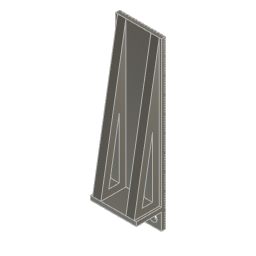
Fixture (Autodesk Fusion 360 design; units mm, degrees)
Autodesk Fusion 360 part; units mm, degrees
(part 1 of 2)
sketch "Sketch1" plane through (0, 0, 0) normal (0, 1, 0) x (1, 0, 0)
  line L0 (0, 0) -> (69.85, 0)
  line L1 (69.85, 0) -> (69.85, -25.4)
  line L2 (69.85, -25.4) -> (0, -25.4)
  line L3 (0, -25.4) -> (0, 0)
  line L4 (4.7498, -25.4) -> (5.5372, -25.4)
  line L5 (5.5372, 0) -> (4.7498, 0)
  line L6 (69.85, -22.225) -> (69.85, -21.4376)
  line L7 (0, -21.4376) -> (0, -22.225)
  line L8 (0, -22.225) -> (4.7498, -22.225)
  line L9 (4.7498, -21.4376) -> (0, -21.4376)
  line L10 (0, -19.05) -> (4.7498, -19.05)
  line L11 (4.7498, -18.2626) -> (0, -18.2626)
  line L12 (0, -15.875) -> (4.7498, -15.875)
  line L13 (4.7498, -15.0876) -> (0, -15.0876)
  line L14 (4.7498, -11.9126) -> (0, -11.9126)
  line L15 (0, -12.7) -> (4.7498, -12.7)
  line L16 (0, -9.525) -> (4.7498, -9.525)
  line L17 (4.7498, -8.7376) -> (0, -8.7376)
  line L18 (0, -6.35) -> (4.7498, -6.35)
  line L19 (4.7498, -5.5626) -> (0, -5.5626)
  line L20 (0, -3.175) -> (4.7498, -3.175)
  line L21 (4.7498, -2.3876) -> (0, -2.3876)
  line L22 (9.4996, -2.3876) -> (5.5372, -2.3876)
  line L23 (5.5372, -3.175) -> (9.4996, -3.175)
  line L24 (9.4996, -5.5626) -> (5.5372, -5.5626)
  line L25 (5.5372, -6.35) -> (9.4996, -6.35)
  line L26 (9.4996, -8.7376) -> (5.5372, -8.7376)
  line L27 (5.5372, -9.525) -> (9.4996, -9.525)
  line L28 (9.4996, -11.9126) -> (5.5372, -11.9126)
  line L29 (5.5372, -12.7) -> (9.4996, -12.7)
  line L30 (9.4996, -15.0876) -> (5.5372, -15.0876)
  line L31 (5.5372, -15.875) -> (9.4996, -15.875)
  line L32 (9.4996, -18.2626) -> (5.5372, -18.2626)
  line L33 (5.5372, -19.05) -> (9.4996, -19.05)
  line L34 (9.4996, -21.4376) -> (5.5372, -21.4376)
  line L35 (5.5372, -22.225) -> (9.4996, -22.225)
  line L36 (10.287, -22.225) -> (14.2494, -22.225)
  line L37 (14.2494, -21.4376) -> (10.287, -21.4376)
  line L38 (10.287, -19.05) -> (14.2494, -19.05)
  line L39 (14.2494, -18.2626) -> (10.287, -18.2626)
  line L40 (10.287, -15.875) -> (14.2494, -15.875)
  line L41 (14.2494, -15.0876) -> (10.287, -15.0876)
  line L42 (10.287, -12.7) -> (14.2494, -12.7)
  line L43 (14.2494, -11.9126) -> (10.287, -11.9126)
  line L44 (10.287, -9.525) -> (14.2494, -9.525)
  line L45 (14.2494, -8.7376) -> (10.287, -8.7376)
  line L46 (10.287, -6.35) -> (14.2494, -6.35)
  line L47 (14.2494, -5.5626) -> (10.287, -5.5626)
  line L48 (10.287, -3.175) -> (14.2494, -3.175)
  line L49 (14.2494, -2.3876) -> (10.287, -2.3876)
  line L50 (18.9992, -2.3876) -> (15.0368, -2.3876)
  line L51 (15.0368, -3.175) -> (18.9992, -3.175)
  line L52 (18.9992, -5.5626) -> (15.0368, -5.5626)
  line L53 (15.0368, -6.35) -> (18.9992, -6.35)
  line L54 (18.9992, -8.7376) -> (15.0368, -8.7376)
  line L55 (15.0368, -9.525) -> (18.9992, -9.525)
  line L56 (18.9992, -11.9126) -> (15.0368, -11.9126)
  line L57 (15.0368, -12.7) -> (18.9992, -12.7)
  line L58 (15.0368, -15.875) -> (18.9992, -15.875)
  line L59 (18.9992, -15.0876) -> (15.0368, -15.0876)
  line L60 (18.9992, -18.2626) -> (15.0368, -18.2626)
  line L61 (15.0368, -19.05) -> (18.9992, -19.05)
  line L62 (18.9992, -21.4376) -> (15.0368, -21.4376)
  line L63 (15.0368, -22.225) -> (18.9992, -22.225)
  line L64 (19.7866, -22.225) -> (23.749, -22.225)
  line L65 (23.749, -21.4376) -> (19.7866, -21.4376)
  line L66 (19.7866, -19.05) -> (23.749, -19.05)
  line L67 (23.749, -18.2626) -> (19.7866, -18.2626)
  line L68 (19.7866, -15.875) -> (23.749, -15.875)
  line L69 (23.749, -15.0876) -> (19.7866, -15.0876)
  line L70 (19.7866, -12.7) -> (23.749, -12.7)
  line L71 (23.749, -11.9126) -> (19.7866, -11.9126)
  line L72 (19.7866, -9.525) -> (23.749, -9.525)
  line L73 (23.749, -8.7376) -> (19.7866, -8.7376)
  line L74 (19.7866, -6.35) -> (23.749, -6.35)
  line L75 (23.749, -5.5626) -> (19.7866, -5.5626)
  line L76 (19.7866, -3.175) -> (23.749, -3.175)
  line L77 (23.749, -2.3876) -> (19.7866, -2.3876)
  line L78 (28.4988, -2.3876) -> (24.5364, -2.3876)
  line L79 (24.5364, -3.175) -> (28.4988, -3.175)
  line L80 (28.4988, -5.5626) -> (24.5364, -5.5626)
  line L81 (24.5364, -6.35) -> (28.4988, -6.35)
  line L82 (28.4988, -8.7376) -> (24.5364, -8.7376)
  line L83 (24.5364, -9.525) -> (28.4988, -9.525)
  line L84 (28.4988, -11.9126) -> (24.5364, -11.9126)
  line L85 (24.5364, -12.7) -> (28.4988, -12.7)
  line L86 (28.4988, -15.0876) -> (24.5364, -15.0876)
  line L87 (24.5364, -15.875) -> (28.4988, -15.875)
  line L88 (28.4988, -18.2626) -> (24.5364, -18.2626)
  line L89 (24.5364, -19.05) -> (28.4988, -19.05)
  line L90 (28.4988, -21.4376) -> (24.5364, -21.4376)
  line L91 (24.5364, -22.225) -> (28.4988, -22.225)
  line L92 (29.2862, -22.225) -> (33.2486, -22.225)
  line L93 (33.2486, -21.4376) -> (29.2862, -21.4376)
  line L94 (29.2862, -19.05) -> (33.2486, -19.05)
  line L95 (33.2486, -18.2626) -> (29.2862, -18.2626)
  line L96 (29.2862, -15.875) -> (33.2486, -15.875)
  line L97 (33.2486, -15.0876) -> (29.2862, -15.0876)
  line L98 (29.2862, -12.7) -> (33.2486, -12.7)
  line L99 (33.2486, -11.9126) -> (29.2862, -11.9126)
  line L100 (29.2862, -9.525) -> (33.2486, -9.525)
  line L101 (33.2486, -8.7376) -> (29.2862, -8.7376)
  line L102 (29.2862, -6.35) -> (33.2486, -6.35)
  line L103 (33.2486, -5.5626) -> (29.2862, -5.5626)
  line L104 (29.2862, -3.175) -> (33.2486, -3.175)
  line L105 (33.2486, -2.3876) -> (29.2862, -2.3876)
  line L106 (37.9984, -2.3876) -> (34.036, -2.3876)
  line L107 (34.036, -3.175) -> (37.9984, -3.175)
  line L108 (37.9984, -5.5626) -> (34.036, -5.5626)
  line L109 (34.036, -6.35) -> (37.9984, -6.35)
  line L110 (37.9984, -8.7376) -> (34.036, -8.7376)
  line L111 (34.036, -9.525) -> (37.9984, -9.525)
  line L112 (37.9984, -11.9126) -> (34.036, -11.9126)
  line L113 (34.036, -12.7) -> (37.9984, -12.7)
  line L114 (37.9984, -15.0876) -> (34.036, -15.0876)
  line L115 (34.036, -15.875) -> (37.9984, -15.875)
  line L116 (37.9984, -18.2626) -> (34.036, -18.2626)
  line L117 (34.036, -19.05) -> (37.9984, -19.05)
  line L118 (37.9984, -21.4376) -> (34.036, -21.4376)
  line L119 (34.036, -22.225) -> (37.9984, -22.225)
  line L120 (38.7858, -22.225) -> (42.7482, -22.225)
  line L121 (42.7482, -21.4376) -> (38.7858, -21.4376)
  line L122 (38.7858, -19.05) -> (42.7482, -19.05)
  line L123 (42.7482, -18.2626) -> (38.7858, -18.2626)
  line L124 (38.7858, -15.875) -> (42.7482, -15.875)
  line L125 (42.7482, -15.0876) -> (38.7858, -15.0876)
  line L126 (38.7858, -12.7) -> (42.7482, -12.7)
  line L127 (42.7482, -11.9126) -> (38.7858, -11.9126)
  line L128 (38.7858, -9.525) -> (42.7482, -9.525)
  line L129 (42.7482, -8.7376) -> (38.7858, -8.7376)
  line L130 (38.7858, -3.175) -> (42.7482, -3.175)
  line L131 (42.7482, -2.3876) -> (38.7858, -2.3876)
  line L132 (42.7482, -5.5626) -> (38.7858, -5.5626)
  line L133 (38.7858, -6.35) -> (42.7482, -6.35)
  line L134 (43.5356, -22.225) -> (47.498, -22.225)
  line L135 (47.498, -21.4376) -> (43.5356, -21.4376)
  line L136 (43.5356, -19.05) -> (47.498, -19.05)
  line L137 (47.498, -18.2626) -> (43.5356, -18.2626)
  line L138 (43.5356, -15.875) -> (47.498, -15.875)
  line L139 (47.498, -15.0876) -> (43.5356, -15.0876)
  line L140 (43.5356, -12.7) -> (47.498, -12.7)
  line L141 (47.498, -11.9126) -> (43.5356, -11.9126)
  line L142 (43.5356, -9.525) -> (47.498, -9.525)
  line L143 (47.498, -8.7376) -> (43.5356, -8.7376)
  line L144 (43.5356, -6.35) -> (47.498, -6.35)
  line L145 (47.498, -5.5626) -> (43.5356, -5.5626)
  line L146 (43.5356, -3.175) -> (47.498, -3.175)
  line L147 (47.498, -2.3876) -> (43.5356, -2.3876)
  line L148 (52.2478, -2.3876) -> (48.2854, -2.3876)
  line L149 (48.2854, -3.175) -> (52.2478, -3.175)
  line L150 (52.2478, -5.5626) -> (48.2854, -5.5626)
  line L151 (48.2854, -6.35) -> (52.2478, -6.35)
  line L152 (52.2478, -8.7376) -> (48.2854, -8.7376)
  line L153 (48.2854, -9.525) -> (52.2478, -9.525)
  line L154 (52.2478, -11.9126) -> (48.2854, -11.9126)
  line L155 (48.2854, -12.7) -> (52.2478, -12.7)
  line L156 (52.2478, -15.0876) -> (48.2854, -15.0876)
  line L157 (48.2854, -15.875) -> (52.2478, -15.875)
  line L158 (52.2478, -18.2626) -> (48.2854, -18.2626)
  line L159 (48.2854, -19.05) -> (52.2478, -19.05)
  line L160 (52.2478, -21.4376) -> (48.2854, -21.4376)
  line L161 (48.2854, -22.225) -> (52.2478, -22.225)
  line L162 (53.0352, -22.225) -> (56.9976, -22.225)
  line L163 (56.9976, -21.4376) -> (53.0352, -21.4376)
  line L164 (53.0352, -19.05) -> (56.9976, -19.05)
  line L165 (56.9976, -18.2626) -> (53.0352, -18.2626)
  line L166 (53.0352, -15.875) -> (56.9976, -15.875)
  line L167 (56.9976, -15.0876) -> (53.0352, -15.0876)
  line L168 (53.0352, -12.7) -> (56.9976, -12.7)
  line L169 (56.9976, -11.9126) -> (53.0352, -11.9126)
  line L170 (53.0352, -9.525) -> (56.9976, -9.525)
  line L171 (56.9976, -9.525) -> (56.9976, -11.9126)
  line L172 (57.785, -11.9126) -> (57.785, -9.525)
  line L173 (56.9976, -8.7376) -> (53.0352, -8.7376)
  line L174 (53.0352, -6.35) -> (56.9976, -6.35)
  line L175 (56.9976, -5.5626) -> (53.0352, -5.5626)
  line L176 (53.0352, -3.175) -> (56.9976, -3.175)
  line L177 (56.9976, -2.3876) -> (53.0352, -2.3876)
  line L178 (61.7474, -2.3876) -> (57.785, -2.3876)
  line L179 (57.785, -3.175) -> (61.7474, -3.175)
  line L180 (61.7474, -5.5626) -> (57.785, -5.5626)
  line L181 (57.785, -6.35) -> (61.7474, -6.35)
  line L182 (61.7474, -8.7376) -> (57.785, -8.7376)
  line L183 (57.785, -9.525) -> (61.7474, -9.525)
  line L184 (61.7474, -11.9126) -> (57.785, -11.9126)
  line L185 (57.785, -12.7) -> (61.7474, -12.7)
  line L186 (61.7474, -15.0876) -> (57.785, -15.0876)
  line L187 (57.785, -15.875) -> (61.7474, -15.875)
  line L188 (61.7474, -18.2626) -> (57.785, -18.2626)
  line L189 (57.785, -19.05) -> (61.7474, -19.05)
  line L190 (61.7474, -21.4376) -> (57.785, -21.4376)
  line L191 (57.785, -22.225) -> (61.7474, -22.225)
  line L192 (62.5348, -22.225) -> (66.4972, -22.225)
  line L193 (67.2846, -22.225) -> (69.85, -22.225)
  line L194 (69.85, -21.4376) -> (67.2846, -21.4376)
  line L195 (66.4972, -21.4376) -> (62.5348, -21.4376)
  line L196 (62.5348, -19.05) -> (66.4972, -19.05)
  line L197 (67.2846, -19.05) -> (69.85, -19.05)
  line L198 (69.85, -18.2626) -> (67.2846, -18.2626)
  line L199 (66.4972, -18.2626) -> (62.5348, -18.2626)
  line L200 (62.5348, -15.875) -> (66.4972, -15.875)
  line L201 (67.2846, -15.875) -> (69.85, -15.875)
  line L202 (69.85, -15.0876) -> (67.2846, -15.0876)
  line L203 (66.4972, -15.0876) -> (62.5348, -15.0876)
  line L204 (62.5348, -12.7) -> (66.4972, -12.7)
  line L205 (67.2846, -12.7) -> (69.85, -12.7)
  line L206 (69.85, -11.9126) -> (67.2846, -11.9126)
  line L207 (66.4972, -11.9126) -> (62.5348, -11.9126)
  line L208 (62.5348, -9.525) -> (66.4972, -9.525)
  line L209 (67.2846, -9.525) -> (69.85, -9.525)
  line L210 (69.85, -8.7376) -> (67.2846, -8.7376)
  line L211 (66.4972, -8.7376) -> (62.5348, -8.7376)
  line L212 (62.5348, -6.35) -> (66.4972, -6.35)
  line L213 (67.2846, -6.35) -> (69.85, -6.35)
  line L214 (69.85, -5.5626) -> (67.2846, -5.5626)
  line L215 (66.4972, -5.5626) -> (62.5348, -5.5626)
  line L216 (62.5348, -3.175) -> (66.4972, -3.175)
  line L217 (67.2846, -3.175) -> (69.85, -3.175)
  line L218 (69.85, -2.3876) -> (67.2846, -2.3876)
  line L219 (66.4972, -2.3876) -> (62.5348, -2.3876)
  line L220 (67.2846, -2.3876) -> (67.2846, 0)
  line L221 (66.4972, 0) -> (66.4972, -2.3876)
  line L222 (62.5348, -2.3876) -> (62.5348, 0)
  line L223 (61.7474, 0) -> (61.7474, -2.3876)
  line L224 (57.785, -2.3876) -> (57.785, 0)
  line L225 (56.9976, 0) -> (56.9976, -2.3876)
  line L226 (56.9976, -3.175) -> (56.9976, -8.7376)
  line L227 (53.0352, -2.3876) -> (53.0352, 0)
  line L228 (52.2478, 0) -> (52.2478, -2.3876)
  line L229 (48.2854, -2.3876) -> (48.2854, 0)
  line L230 (47.498, 0) -> (47.498, -2.3876)
  line L231 (43.5356, -2.3876) -> (43.5356, 0)
  line L232 (42.7482, 0) -> (42.7482, -2.3876)
  line L233 (38.7858, -2.3876) -> (38.7858, 0)
  line L234 (37.9984, 0) -> (37.9984, -2.3876)
  line L235 (34.036, -2.3876) -> (34.036, 0)
  line L236 (33.2486, 0) -> (33.2486, -2.3876)
  line L237 (29.2862, -2.3876) -> (29.2862, 0)
  line L238 (28.4988, 0) -> (28.4988, -2.3876)
  line L239 (24.5364, -2.3876) -> (24.5364, 0)
  line L240 (23.749, 0) -> (23.749, -2.3876)
  line L241 (19.7866, -2.3876) -> (19.7866, 0)
  line L242 (18.9992, 0) -> (18.9992, -2.3876)
  line L243 (15.0368, -2.3876) -> (15.0368, 0)
  line L244 (14.2494, 0) -> (14.2494, -2.3876)
  line L245 (10.287, -2.3876) -> (10.287, 0)
  line L246 (5.5372, -2.3876) -> (5.5372, 0)
  line L247 (4.7498, 0) -> (4.7498, -2.3876)
  line L248 (9.4996, 0) -> (9.4996, -2.3876)
  line L249 (9.4996, -3.175) -> (9.4996, -5.5626)
  line L250 (5.5372, -5.5626) -> (5.5372, -3.175)
  line L251 (4.7498, -3.175) -> (4.7498, -5.5626)
  line L252 (10.287, -5.5626) -> (10.287, -3.175)
  line L253 (15.0368, -5.5626) -> (15.0368, -3.175)
  line L254 (18.9992, -3.175) -> (18.9992, -5.5626)
  line L255 (19.7866, -5.5626) -> (19.7866, -3.175)
  line L256 (24.5364, -5.5626) -> (24.5364, -3.175)
  line L257 (29.2862, -5.5626) -> (29.2862, -3.175)
  line L258 (28.4988, -3.175) -> (28.4988, -5.5626)
  line L259 (23.749, -3.175) -> (23.749, -5.5626)
  line L260 (33.2486, -3.175) -> (33.2486, -5.5626)
  line L261 (33.2486, -6.35) -> (33.2486, -8.7376)
  line L262 (34.036, -5.5626) -> (34.036, -3.175)
  line L263 (37.9984, -3.175) -> (37.9984, -5.5626)
  line L264 (38.7858, -5.5626) -> (38.7858, -3.175)
  line L265 (42.7482, -3.175) -> (42.7482, -5.5626)
  line L266 (43.5356, -5.5626) -> (43.5356, -3.175)
  line L267 (47.498, -3.175) -> (47.498, -5.5626)
  line L268 (48.2854, -5.5626) -> (48.2854, -3.175)
  line L269 (52.2478, -3.175) -> (52.2478, -5.5626)
  line L270 (53.0352, -5.5626) -> (53.0352, -3.175)
  line L271 (57.785, -8.7376) -> (57.785, -6.35)
  line L272 (57.785, -5.5626) -> (57.785, -3.175)
  line L273 (61.7474, -3.175) -> (61.7474, -5.5626)
  line L274 (62.5348, -5.5626) -> (62.5348, -3.175)
  line L275 (66.4972, -3.175) -> (66.4972, -5.5626)
  line L276 (67.2846, -5.5626) -> (67.2846, -3.175)
  line L277 (67.2846, -8.7376) -> (67.2846, -6.35)
  line L278 (66.4972, -6.35) -> (66.4972, -8.7376)
  line L279 (62.5348, -8.7376) -> (62.5348, -6.35)
  line L280 (61.7474, -6.35) -> (61.7474, -8.7376)
  line L281 (53.0352, -8.7376) -> (53.0352, -6.35)
  line L282 (52.2478, -6.35) -> (52.2478, -8.7376)
  line L283 (48.2854, -8.7376) -> (48.2854, -6.35)
  line L284 (47.498, -6.35) -> (47.498, -8.7376)
  line L285 (43.5356, -8.7376) -> (43.5356, -6.35)
  line L286 (42.7482, -6.35) -> (42.7482, -8.7376)
  line L287 (38.7858, -8.7376) -> (38.7858, -6.35)
  line L288 (37.9984, -6.35) -> (37.9984, -8.7376)
  line L289 (34.036, -8.7376) -> (34.036, -6.35)
  line L290 (29.2862, -8.7376) -> (29.2862, -6.35)
  line L291 (28.4988, -6.35) -> (28.4988, -8.7376)
  line L292 (24.5364, -8.7376) -> (24.5364, -6.35)
  line L293 (23.749, -6.35) -> (23.749, -8.7376)
  line L294 (19.7866, -8.7376) -> (19.7866, -6.35)
  line L295 (18.9992, -6.35) -> (18.9992, -8.7376)
  line L296 (15.0368, -8.7376) -> (15.0368, -6.35)
  line L297 (14.2494, -3.175) -> (14.2494, -8.7376)
  line L298 (9.4996, -6.35) -> (9.4996, -8.7376)
  line L299 (4.7498, -6.35) -> (4.7498, -8.7376)
  line L300 (4.7498, -11.9126) -> (4.7498, -9.525)
  line L301 (10.287, -6.35) -> (10.287, -8.7376)
  line L302 (5.5372, -8.7376) -> (5.5372, -6.35)
  line L303 (67.2846, -11.9126) -> (67.2846, -9.525)
  line L304 (66.4972, -9.525) -> (66.4972, -15.0876)
  line L305 (67.2846, -15.0876) -> (67.2846, -12.7)
  line L306 (61.7474, -9.525) -> (61.7474, -11.9126)
  line L307 (61.7474, -12.7) -> (61.7474, -15.0876)
  line L308 (62.5348, -15.0876) -> (62.5348, -12.7)
  line L309 (62.5348, -11.9126) -> (62.5348, -9.525)
  line L310 (57.785, -15.0876) -> (57.785, -12.7)
  line L311 (53.0352, -11.9126) -> (53.0352, -9.525)
  line L312 (53.0352, -15.0876) -> (53.0352, -12.7)
  line L313 (56.9976, -12.7) -> (56.9976, -15.0876)
  line L314 (52.2478, -9.525) -> (52.2478, -11.9126)
  line L315 (52.2478, -12.7) -> (52.2478, -15.0876)
  line L316 (48.2854, -15.0876) -> (48.2854, -12.7)
  line L317 (48.2854, -11.9126) -> (48.2854, -9.525)
  line L318 (47.498, -15.875) -> (47.498, -25.4)
  line L319 (47.498, -9.525) -> (47.498, -11.9126)
  line L320 (47.498, -12.7) -> (47.498, -15.0876)
  line L321 (43.5356, -15.0876) -> (43.5356, -12.7)
  line L322 (43.5356, -11.9126) -> (43.5356, -9.525)
  line L323 (42.7482, -9.525) -> (42.7482, -11.9126)
  line L324 (42.7482, -12.7) -> (42.7482, -15.0876)
  line L325 (38.7858, -11.9126) -> (38.7858, -9.525)
  line L326 (37.9984, -9.525) -> (37.9984, -11.9126)
  line L327 (38.7858, -15.0876) -> (38.7858, -12.7)
  line L328 (33.2486, -9.525) -> (33.2486, -11.9126)
  line L329 (33.2486, -12.7) -> (33.2486, -15.0876)
  line L330 (34.036, -15.0876) -> (34.036, -12.7)
  line L331 (34.036, -11.9126) -> (34.036, -9.525)
  line L332 (28.4988, -9.525) -> (28.4988, -11.9126)
  line L333 (28.4988, -12.7) -> (28.4988, -15.0876)
  line L334 (29.2862, -15.0876) -> (29.2862, -12.7)
  line L335 (29.2862, -11.9126) -> (29.2862, -9.525)
  line L336 (37.9984, -12.7) -> (37.9984, -15.0876)
  line L337 (24.5364, -11.9126) -> (24.5364, -9.525)
  line L338 (23.749, -9.525) -> (23.749, -11.9126)
  line L339 (23.749, -12.7) -> (23.749, -15.0876)
  line L340 (24.5364, -15.0876) -> (24.5364, -12.7)
  line L341 (19.7866, -15.0876) -> (19.7866, -12.7)
  line L342 (19.7866, -11.9126) -> (19.7866, -9.525)
  line L343 (18.9992, -9.525) -> (18.9992, -11.9126)
  line L344 (18.9992, -12.7) -> (18.9992, -15.0876)
  line L345 (14.2494, -9.525) -> (14.2494, -11.9126)
  line L346 (14.2494, -12.7) -> (14.2494, -15.0876)
  line L347 (15.0368, -15.0876) -> (15.0368, -12.7)
  line L348 (15.0368, -11.9126) -> (15.0368, -9.525)
  line L349 (10.287, -11.9126) -> (10.287, -9.525)
  line L350 (9.4996, -9.525) -> (9.4996, -11.9126)
  line L351 (9.4996, -12.7) -> (9.4996, -15.0876)
  line L352 (10.287, -15.0876) -> (10.287, -12.7)
  line L353 (4.7498, -12.7) -> (4.7498, -15.0876)
  line L354 (5.5372, -15.0876) -> (5.5372, -12.7)
  line L355 (5.5372, -11.9126) -> (5.5372, -9.525)
  line L356 (4.7498, -22.225) -> (4.7498, -25.4)
  line L357 (5.5372, -25.4) -> (5.5372, -22.225)
  line L358 (4.7498, -15.875) -> (4.7498, -18.2626)
  line L359 (4.7498, -19.05) -> (4.7498, -21.4376)
  line L360 (5.5372, -21.4376) -> (5.5372, -19.05)
  line L361 (5.5372, -18.2626) -> (5.5372, -15.875)
  line L362 (9.4996, -22.225) -> (9.4996, -25.4)
  line L363 (9.4996, -15.875) -> (9.4996, -18.2626)
  line L364 (9.4996, -19.05) -> (9.4996, -21.4376)
  line L365 (10.287, -18.2626) -> (10.287, -15.875)
  line L366 (10.287, -25.4) -> (10.287, -22.225)
  line L367 (10.287, -21.4376) -> (10.287, -19.05)
  line L368 (14.2494, -22.225) -> (14.2494, -25.4)
  line L369 (14.2494, -15.875) -> (14.2494, -18.2626)
  line L370 (14.2494, -19.05) -> (14.2494, -21.4376)
  line L371 (15.0368, -25.4) -> (15.0368, -22.225)
  line L372 (15.0368, -21.4376) -> (15.0368, -19.05)
  line L373 (15.0368, -18.2626) -> (15.0368, -15.875)
  line L374 (18.9992, -15.875) -> (18.9992, -18.2626)
  line L375 (18.9992, -19.05) -> (18.9992, -21.4376)
  line L376 (18.9992, -22.225) -> (18.9992, -25.4)
  line L377 (19.7866, -25.4) -> (19.7866, -22.225)
  line L378 (19.7866, -21.4376) -> (19.7866, -19.05)
  line L379 (19.7866, -18.2626) -> (19.7866, -15.875)
  line L380 (23.749, -22.225) -> (23.749, -25.4)
  line L381 (24.5364, -25.4) -> (24.5364, -22.225)
  line L382 (23.749, -15.875) -> (23.749, -18.2626)
  line L383 (23.749, -19.05) -> (23.749, -21.4376)
  line L384 (24.5364, -21.4376) -> (24.5364, -19.05)
  line L385 (24.5364, -18.2626) -> (24.5364, -15.875)
  line L386 (29.2862, -25.4) -> (29.2862, -22.225)
  line L387 (28.4988, -22.225) -> (28.4988, -25.4)
  line L388 (28.4988, -15.875) -> (28.4988, -18.2626)
  line L389 (28.4988, -19.05) -> (28.4988, -21.4376)
  line L390 (29.2862, -21.4376) -> (29.2862, -19.05)
  line L391 (29.2862, -18.2626) -> (29.2862, -15.875)
  line L392 (33.2486, -22.225) -> (33.2486, -25.4)
  line L393 (34.036, -25.4) -> (34.036, -22.225)
  line L394 (33.2486, -15.875) -> (33.2486, -18.2626)
  line L395 (33.2486, -19.05) -> (33.2486, -21.4376)
  line L396 (34.036, -21.4376) -> (34.036, -19.05)
  line L397 (34.036, -18.2626) -> (34.036, -15.875)
  line L398 (37.9984, -22.225) -> (37.9984, -25.4)
  line L399 (38.7858, -25.4) -> (38.7858, -22.225)
  line L400 (38.7858, -21.4376) -> (38.7858, -19.05)
  line L401 (38.7858, -18.2626) -> (38.7858, -15.875)
  line L402 (37.9984, -15.875) -> (37.9984, -18.2626)
  line L403 (37.9984, -19.05) -> (37.9984, -21.4376)
  line L404 (43.5356, -25.4) -> (43.5356, -22.225)
  line L405 (42.7482, -22.225) -> (42.7482, -25.4)
  line L406 (42.7482, -15.875) -> (42.7482, -18.2626)
  line L407 (42.7482, -19.05) -> (42.7482, -21.4376)
  line L408 (43.5356, -21.4376) -> (43.5356, -19.05)
  line L409 (43.5356, -18.2626) -> (43.5356, -15.875)
  line L410 (48.2854, -25.4) -> (48.2854, -22.225)
  line L411 (52.2478, -22.225) -> (52.2478, -25.4)
  line L412 (53.0352, -25.4) -> (53.0352, -22.225)
  line L413 (53.0352, -21.4376) -> (53.0352, -19.05)
  line L414 (53.0352, -18.2626) -> (53.0352, -15.875)
  line L415 (52.2478, -15.875) -> (52.2478, -18.2626)
  line L416 (52.2478, -19.05) -> (52.2478, -21.4376)
  line L417 (48.2854, -21.4376) -> (48.2854, -19.05)
  line L418 (48.2854, -18.2626) -> (48.2854, -15.875)
  line L419 (56.9976, -15.875) -> (56.9976, -18.2626)
  line L420 (56.9976, -19.05) -> (56.9976, -21.4376)
  line L421 (56.9976, -22.225) -> (56.9976, -25.4)
  line L422 (57.785, -25.4) -> (57.785, -22.225)
  line L423 (57.785, -21.4376) -> (57.785, -19.05)
  line L424 (57.785, -18.2626) -> (57.785, -15.875)
  line L425 (61.7474, -15.875) -> (61.7474, -18.2626)
  line L426 (61.7474, -19.05) -> (61.7474, -21.4376)
  line L427 (61.7474, -22.225) -> (61.7474, -25.4)
  line L428 (62.5348, -25.4) -> (62.5348, -22.225)
  line L429 (62.5348, -21.4376) -> (62.5348, -19.05)
  line L430 (62.5348, -18.2626) -> (62.5348, -15.875)
  line L431 (66.4972, -22.225) -> (66.4972, -25.4)
  line L432 (67.2846, -25.4) -> (67.2846, -22.225)
  line L433 (66.4972, -15.875) -> (66.4972, -18.2626)
  line L434 (66.4972, -19.05) -> (66.4972, -21.4376)
  line L435 (67.2846, -21.4376) -> (67.2846, -19.05)
  line L436 (67.2846, -18.2626) -> (67.2846, -15.875)
  point P0 (12.7, -12.7)
  point P1 (57.15, -12.7)
  dimension "d1" = 69.85
  dimension "d2" = 25.4
  dimension "d3" = 0.7874
  dimension "d4" = 4.7498
  dimension "d9" = 0.7874
  dimension "d10" = 3.175
  dimension "d15" = 12.7
  dimension "d16" = 12.7
  dimension "d17" = 12.7
  dimension "d18" = 12.7
  constraint horizontal L0
  constraint vertical L1
  constraint horizontal L2
  constraint vertical L3
  constraint coincident L0.start L3.end
  constraint horizontal L4
  constraint vertical L357
  constraint horizontal L5
  constraint vertical L247
  constraint coincident L2 L4.start
  constraint horizontal L8
  constraint vertical L6
  constraint horizontal L194
  constraint vertical L7
  constraint coincident L8.end L247
  constraint collinear L8 L35
  constraint coincident L34.end L357
  constraint coincident L9.start L247
  constraint collinear L9 L194
  constraint coincident L10.end L247
  constraint coincident L33.start L357
  constraint collinear L10 L33
  constraint coincident L32.end L357
  constraint coincident L11.start L247
  constraint collinear L11 L198
  constraint coincident L12.end L247
  constraint collinear L12 L31
  constraint coincident L30.end L357
  constraint coincident L13.start L247
  constraint collinear L13 L202
  constraint coincident L28.end L357
  constraint coincident L14.start L247
  constraint collinear L14 L206
  constraint coincident L15.end L247
  constraint coincident L29.start L357
  constraint collinear L15 L29
  constraint coincident L16.end L247
  constraint collinear L16 L27
  constraint coincident L26.end L357
  constraint coincident L17.start L247
  constraint collinear L17 L210
  constraint coincident L18.end L247
  constraint collinear L18 L25
  constraint coincident L24.end L357
  constraint coincident L19.start L247
  constraint collinear L19 L214
  constraint coincident L20.end L247
  constraint collinear L20 L23
  constraint coincident L22.end L357
  constraint collinear L21 L218
  constraint coincident L49.end L366
  constraint collinear L22 L218
  constraint coincident L23.end L248
  constraint collinear L23 L48
  constraint coincident L47.end L366
  constraint coincident L24.start L248
  constraint collinear L24 L214
  constraint coincident L25.end L248
  constraint collinear L25 L46
  constraint coincident L26.start L248
  constraint collinear L26 L210
  constraint coincident L27.end L248
  constraint collinear L27 L44
  constraint coincident L43.end L366
  constraint coincident L28.start L248
  constraint collinear L28 L206
  constraint coincident L29.end L248
  constraint collinear L29 L42
  constraint coincident L41.end L366
  constraint coincident L30.start L248
  constraint collinear L30 L202
  constraint coincident L31.end L248
  constraint collinear L31 L40
  constraint coincident L39.end L366
  constraint coincident L32.start L248
  constraint collinear L32 L198
  constraint coincident L33.end L248
  constraint collinear L33 L38
  constraint coincident L37.end L366
  constraint coincident L34.start L248
  constraint collinear L34 L194
  constraint coincident L35.end L248
  constraint collinear L35 L36
  constraint coincident L36.end L244
  constraint collinear L36 L63
  constraint coincident L62.end L371
  constraint coincident L37.start L244
  constraint collinear L37 L194
  constraint coincident L38.end L244
  constraint coincident L61.start L371
  constraint collinear L38 L61
  constraint coincident L60.end L371
  constraint coincident L39.start L244
  constraint collinear L39 L198
  constraint coincident L40.end L244
  constraint collinear L40 L58
  constraint coincident L59.end L371
  constraint coincident L41.start L244
  constraint collinear L41 L202
  constraint coincident L42.end L244
  constraint coincident L57.start L371
  constraint collinear L42 L57
  constraint coincident L56.end L371
  constraint coincident L43.start L244
  constraint collinear L43 L206
  constraint coincident L44.end L244
  constraint collinear L44 L55
  constraint coincident L54.end L371
  constraint coincident L45.start L244
  constraint collinear L45 L210
  constraint coincident L46.end L244
  constraint collinear L46 L53
  constraint coincident L52.end L371
  constraint coincident L47.start L244
  constraint collinear L47 L214
  constraint coincident L48.end L244
  constraint collinear L48 L51
  constraint coincident L50.end L371
  constraint collinear L49 L218
  constraint coincident L77.end L377
  constraint collinear L50 L218
  constraint coincident L51.end L242
  constraint collinear L51 L76
  constraint coincident L75.end L377
  constraint coincident L52.start L242
  constraint collinear L52 L214
  constraint coincident L53.end L242
  constraint collinear L53 L74
  constraint coincident L73.end L377
  constraint coincident L54.start L242
  constraint collinear L54 L210
  constraint coincident L55.end L242
  constraint collinear L55 L72
  constraint coincident L71.end L377
  constraint coincident L56.start L242
  constraint collinear L56 L206
  constraint coincident L57.end L242
  constraint coincident L70.start L377
  constraint collinear L57 L70
  constraint coincident L58.end L242
  constraint collinear L58 L68
  constraint coincident L69.end L377
  constraint coincident L59.start L242
  constraint collinear L59 L202
  constraint coincident L67.end L377
  constraint coincident L60.start L242
  constraint collinear L60 L198
  constraint coincident L61.end L242
  constraint coincident L66.start L377
  constraint collinear L61 L66
  constraint coincident L65.end L377
  constraint coincident L62.start L242
  constraint collinear L62 L194
  constraint coincident L63.end L242
  constraint collinear L63 L64
  constraint coincident L64.end L240
  constraint collinear L64 L91
  constraint coincident L90.end L381
  constraint coincident L65.start L240
  constraint collinear L65 L194
  constraint coincident L66.end L240
  constraint coincident L89.start L381
  constraint collinear L66 L89
  constraint coincident L88.end L381
  constraint coincident L67.start L240
  constraint collinear L67 L198
  constraint coincident L68.end L240
  constraint collinear L68 L87
  constraint coincident L86.end L381
  constraint coincident L69.start L240
  constraint collinear L69 L202
  constraint coincident L70.end L240
  constraint collinear L70 L85
  constraint coincident L84.end L381
  constraint coincident L71.start L240
  constraint collinear L71 L206
  constraint coincident L72.end L240
  constraint collinear L72 L83
  constraint coincident L82.end L381
  constraint coincident L73.start L240
  constraint collinear L73 L210
  constraint coincident L74.end L240
  constraint collinear L74 L81
  constraint coincident L80.end L381
  constraint coincident L75.start L240
  constraint collinear L75 L214
  constraint coincident L76.end L240
  constraint collinear L76 L79
  constraint coincident L78.end L381
  constraint collinear L77 L218
  constraint coincident L105.end L386
  constraint collinear L78 L218
  constraint coincident L79.end L238
  constraint collinear L79 L104
  constraint coincident L103.end L386
  constraint coincident L80.start L238
  constraint collinear L80 L214
  constraint coincident L81.end L238
  constraint collinear L81 L102
  constraint coincident L101.end L386
  constraint coincident L82.start L238
  constraint collinear L82 L210
  constraint coincident L83.end L238
  constraint collinear L83 L100
  constraint coincident L99.end L386
  constraint coincident L84.start L238
  constraint collinear L84 L206
  constraint coincident L85.end L238
  constraint coincident L98.start L386
  constraint collinear L85 L98
  constraint coincident L97.end L386
  constraint coincident L86.start L238
  constraint collinear L86 L202
  constraint coincident L87.end L238
  constraint collinear L87 L96
  constraint coincident L95.end L386
  constraint coincident L88.start L238
  constraint collinear L88 L198
  constraint coincident L89.end L238
  constraint coincident L94.start L386
  constraint collinear L89 L94
  constraint coincident L93.end L386
  constraint coincident L90.start L238
  constraint collinear L90 L194
  constraint coincident L91.end L238
  constraint collinear L91 L92
  constraint coincident L92.end L236
  constraint collinear L92 L119
  constraint coincident L118.end L393
  constraint coincident L93.start L236
  constraint collinear L93 L194
  constraint coincident L94.end L236
  constraint coincident L117.start L393
  constraint collinear L94 L117
  constraint coincident L116.end L393
  constraint coincident L95.start L236
  constraint collinear L95 L198
  constraint coincident L96.end L236
  constraint collinear L96 L115
  constraint coincident L114.end L393
  constraint coincident L97.start L236
  constraint collinear L97 L202
  constraint coincident L98.end L236
  constraint coincident L113.start L393
  constraint collinear L98 L113
  constraint coincident L112.end L393
  constraint coincident L99.start L236
  constraint collinear L99 L206
  constraint coincident L100.end L236
  constraint collinear L100 L111
  constraint coincident L101.start L210
  constraint collinear L236 L328
  constraint coincident L110.end L393
  constraint collinear L101 L210
  constraint coincident L102.end L236
  constraint collinear L102 L109
  constraint coincident L108.end L393
  constraint coincident L103.start L236
  constraint collinear L103 L214
  constraint coincident L104.end L236
  constraint collinear L104 L107
  constraint coincident L106.end L393
  constraint collinear L105 L218
  constraint coincident L131.end L399
  constraint collinear L106 L218
  constraint coincident L107.end L234
  constraint collinear L107 L130
  constraint coincident L132.end L399
  constraint coincident L108.start L234
  constraint collinear L108 L214
  constraint coincident L109.end L234
  constraint collinear L109 L133
  constraint coincident L129.end L399
  constraint coincident L110.start L234
  constraint collinear L110 L210
  constraint coincident L111.end L234
  constraint collinear L111 L128
  constraint coincident L127.end L399
  constraint coincident L112.start L234
  constraint collinear L112 L206
  constraint coincident L113.end L234
  constraint collinear L113 L126
  constraint coincident L125.end L399
  constraint coincident L114.start L234
  constraint collinear L114 L202
  constraint coincident L115.end L234
  constraint collinear L115 L124
  constraint coincident L123.end L399
  constraint coincident L116.start L234
  constraint collinear L116 L198
  constraint coincident L117.end L234
  constraint coincident L122.start L399
  constraint collinear L117 L122
  constraint coincident L121.end L399
  constraint coincident L118.start L234
  constraint collinear L118 L194
  constraint coincident L119.end L234
  constraint collinear L119 L120
  constraint coincident L120.end L232
  constraint collinear L120 L134
  constraint coincident L135.end L404
  constraint coincident L121.start L232
  constraint collinear L121 L194
  constraint coincident L122.end L232
  constraint coincident L136.start L404
  constraint collinear L122 L136
  constraint coincident L137.end L404
  constraint coincident L123.start L232
  constraint collinear L123 L198
  constraint coincident L124.end L232
  constraint collinear L124 L138
  constraint coincident L139.end L404
  constraint coincident L125.start L232
  constraint collinear L125 L202
  constraint coincident L126.end L232
  constraint coincident L140.start L404
  constraint collinear L126 L140
  constraint coincident L141.end L404
  constraint coincident L127.start L232
  constraint collinear L127 L206
  constraint coincident L128.end L232
  constraint collinear L128 L142
  constraint coincident L143.end L404
  constraint coincident L129.start L232
  constraint collinear L129 L210
  constraint coincident L130.end L232
  constraint collinear L130 L146
  constraint coincident L147.end L404
  constraint collinear L131 L218
  constraint coincident L145.end L404
  constraint coincident L132.start L232
  constraint collinear L132 L214
  constraint coincident L133.end L232
  constraint collinear L133 L144
  constraint coincident L134.end L230
  constraint collinear L134 L161
  constraint coincident L160.end L410
  constraint coincident L135.start L230
  constraint collinear L135 L194
  constraint coincident L136.end L230
  constraint coincident L159.start L410
  constraint collinear L136 L159
  constraint coincident L158.end L410
  constraint coincident L137.start L230
  constraint collinear L137 L198
  constraint coincident L138.end L230
  constraint collinear L138 L157
  constraint coincident L156.end L410
  constraint coincident L139.start L230
  constraint collinear L139 L202
  constraint coincident L140.end L230
  constraint coincident L155.start L410
  constraint collinear L140 L155
  constraint coincident L154.end L410
  constraint coincident L141.start L230
  constraint collinear L141 L206
  constraint coincident L142.end L230
  constraint collinear L142 L153
  constraint coincident L152.end L410
  constraint coincident L143.start L230
  constraint collinear L143 L210
  constraint coincident L144.end L230
  constraint collinear L144 L151
  constraint coincident L150.end L410
  constraint coincident L145.start L230
  constraint collinear L145 L214
  constraint coincident L146.end L230
  constraint collinear L146 L149
  constraint coincident L148.end L410
  constraint collinear L147 L218
  constraint coincident L177.end L412
  constraint collinear L148 L218
  constraint coincident L149.end L228
  constraint collinear L149 L176
  constraint coincident L175.end L412
  constraint coincident L150.start L228
  constraint collinear L150 L214
  constraint coincident L151.end L228
  constraint collinear L151 L174
  constraint coincident L173.end L412
  constraint coincident L152.start L228
  constraint collinear L152 L210
  constraint coincident L153.end L228
  constraint collinear L153 L170
  constraint coincident L169.end L412
  constraint coincident L154.start L228
  constraint collinear L154 L206
  constraint coincident L155.end L228
  constraint collinear L155 L168
  constraint coincident L167.end L412
  constraint coincident L156.start L228
  constraint collinear L156 L202
  constraint coincident L157.end L228
  constraint collinear L157 L166
  constraint coincident L165.end L412
  constraint coincident L158.start L228
  constraint collinear L158 L198
  constraint coincident L159.end L228
  constraint coincident L164.start L412
  constraint collinear L159 L164
  constraint coincident L163.end L412
  constraint coincident L160.start L228
  constraint collinear L160 L194
  constraint coincident L161.end L228
  constraint collinear L161 L162
  constraint coincident L162.end L225
  constraint collinear L162 L191
  constraint coincident L190.end L422
  constraint coincident L163.start L225
  constraint collinear L163 L194
  constraint coincident L164.end L225
  constraint coincident L189.start L422
  constraint collinear L164 L189
  constraint coincident L188.end L422
  constraint coincident L165.start L225
  constraint collinear L165 L198
  constraint coincident L166.end L225
  constraint collinear L166 L187
  constraint coincident L186.end L422
  constraint coincident L167.start L225
  constraint collinear L167 L202
  constraint coincident L169.start L206
  constraint collinear L225 L313
  constraint collinear L168 L185
  constraint coincident L172.start L422
  constraint collinear L169 L206
  constraint collinear L172 L422
  constraint coincident L170.end L225
  constraint collinear L170 L183
  constraint coincident L173.start L210
  constraint collinear L171 L225
  constraint collinear L172 L271
  constraint collinear L173 L210
  constraint coincident L174.end L225
  constraint collinear L174 L181
  constraint coincident L180.end L271
  constraint coincident L175.start L225
  constraint collinear L175 L214
  constraint coincident L176.end L225
  constraint collinear L176 L179
  constraint coincident L178.end L271
  constraint collinear L177 L218
  constraint coincident L219.end L428
  constraint collinear L178 L218
  constraint coincident L179.end L223
  constraint collinear L179 L216
  constraint coincident L215.end L428
  constraint coincident L180.start L223
  constraint collinear L180 L214
  constraint coincident L181.end L223
  constraint collinear L181 L212
  constraint coincident L211.end L428
  constraint coincident L182.start L223
  constraint collinear L182 L210
  constraint coincident L183.end L223
  constraint collinear L183 L208
  constraint coincident L207.end L428
  constraint coincident L184.start L223
  constraint collinear L184 L206
  constraint coincident L185.end L223
  constraint coincident L204.start L428
  constraint collinear L185 L204
  constraint coincident L203.end L428
  constraint coincident L186.start L223
  constraint collinear L186 L202
  constraint coincident L187.end L223
  constraint collinear L187 L200
  constraint coincident L199.end L428
  constraint coincident L188.start L223
  constraint collinear L188 L198
  constraint coincident L189.end L223
  constraint coincident L196.start L428
  constraint collinear L189 L196
  constraint coincident L195.end L428
  constraint coincident L190.start L223
  constraint collinear L190 L194
  constraint coincident L191.end L223
  constraint collinear L191 L192
  constraint coincident L192.end L221
  constraint collinear L192 L193
  constraint coincident L194.end L432
  constraint coincident L195.start L221
  constraint collinear L194 L195
  constraint coincident L196.end L221
  constraint coincident L197.start L432
  constraint collinear L196 L197
  constraint coincident L198.end L432
  constraint coincident L199.start L221
  constraint collinear L198 L199
  constraint coincident L200.end L221
  constraint collinear L200 L201
  constraint coincident L202.end L432
  constraint coincident L203.start L221
  constraint collinear L202 L203
  constraint coincident L204.end L221
  constraint collinear L204 L205
  constraint coincident L206.end L432
  constraint coincident L207.start L221
  constraint collinear L206 L207
  constraint coincident L208.end L221
  constraint collinear L208 L209
  constraint coincident L210.end L432
  constraint coincident L211.start L221
  constraint collinear L210 L211
  constraint coincident L212.end L221
  constraint collinear L212 L213
  constraint coincident L214.end L432
  constraint coincident L215.start L221
  constraint collinear L214 L215
  constraint coincident L216.end L221
  constraint collinear L216 L217
  constraint coincident L218.end L432
  constraint collinear L218 L219
  constraint collinear L220 L432
  constraint collinear L221 L275
  constraint collinear L222 L428
  constraint collinear L223 L273
  constraint collinear L224 L271
  constraint collinear L225 L226
  constraint collinear L227 L412
  constraint collinear L228 L269
  constraint collinear L229 L410
  constraint collinear L230 L267
  constraint collinear L231 L404
  constraint collinear L232 L265
  constraint collinear L233 L399
  constraint collinear L234 L263
  constraint collinear L235 L393
  constraint collinear L236 L260
  constraint collinear L237 L386
  constraint collinear L238 L258
  constraint collinear L239 L381
  constraint collinear L240 L259
  constraint collinear L241 L377
  constraint collinear L242 L254
  constraint collinear L243 L371
  constraint collinear L244 L297
  constraint collinear L245 L366
  constraint collinear L246 L357
  constraint collinear L247 L251
  constraint collinear L248 L249
  constraint collinear L249 L298
  constraint collinear L250 L357
  constraint collinear L251 L299
  constraint collinear L252 L366
  constraint collinear L253 L371
  constraint collinear L254 L295
  constraint collinear L255 L377
  constraint collinear L256 L381
  constraint collinear L257 L386
  constraint collinear L258 L291
  constraint collinear L259 L293
  constraint collinear L260 L261
  constraint collinear L262 L393
  constraint collinear L263 L288
  constraint collinear L264 L399
  constraint collinear L265 L286
  constraint collinear L266 L404
  constraint collinear L267 L284
  constraint collinear L268 L410
  constraint collinear L269 L282
  constraint collinear L270 L412
  constraint collinear L271 L272
  constraint collinear L273 L280
  constraint collinear L274 L428
  constraint collinear L275 L278
  constraint collinear L276 L432
  constraint collinear L277 L432
  constraint collinear L278 L304
  constraint collinear L279 L428
  constraint collinear L280 L306
  constraint collinear L281 L412
  constraint collinear L282 L314
  constraint collinear L283 L410
  constraint collinear L284 L319
  constraint collinear L285 L404
  constraint collinear L286 L323
  constraint collinear L287 L399
  constraint collinear L288 L326
  constraint collinear L289 L393
  constraint collinear L290 L386
  constraint collinear L291 L332
  constraint collinear L292 L381
  constraint collinear L293 L338
  constraint collinear L294 L377
  constraint collinear L295 L343
  constraint collinear L296 L371
  constraint collinear L297 L345
  constraint collinear L298 L350
  constraint collinear L299 L353
  constraint perpendicular L16 L300
  constraint perpendicular L45 L301
  constraint collinear L302 L357
  constraint collinear L303 L432
  constraint collinear L304 L433
  constraint collinear L305 L432
  constraint collinear L308 L428
  constraint collinear L306 L425
  constraint collinear L306 L307
  constraint collinear L308 L309
  constraint collinear L310 L422
  constraint collinear L311 L412
  constraint collinear L312 L412
  constraint collinear L313 L419
  constraint collinear L314 L315
  constraint collinear L315 L415
  constraint collinear L316 L410
  constraint collinear L316 L317
  constraint collinear L318 L319
  constraint collinear L319 L320
  constraint collinear L323 L406
  constraint collinear L321 L404
  constraint collinear L321 L322
  constraint collinear L323 L324
  constraint collinear L325 L399
  constraint collinear L326 L336
  constraint collinear L327 L399
  constraint collinear L330 L393
  constraint collinear L328 L394
  constraint collinear L328 L329
  constraint collinear L330 L331
  constraint collinear L334 L386
  constraint collinear L332 L388
  constraint collinear L332 L333
  constraint collinear L334 L335
  constraint collinear L336 L402
  constraint collinear L337 L381
  constraint collinear L338 L339
  constraint collinear L339 L382
  constraint collinear L340 L381
  constraint collinear L341 L377
  constraint collinear L341 L342
  constraint collinear L343 L344
  constraint collinear L344 L374
  constraint collinear L347 L371
  constraint collinear L345 L369
  constraint collinear L345 L346
  constraint collinear L347 L348
  constraint collinear L349 L366
  constraint collinear L350 L351
  constraint collinear L351 L363
  constraint collinear L352 L366
  constraint collinear L354 L357
  constraint collinear L353 L358
  constraint collinear L354 L355
  constraint collinear L356 L358
  constraint collinear L357 L360
  constraint collinear L358 L359
  constraint collinear L360 L361
  constraint collinear L362 L363
  constraint collinear L363 L364
  constraint collinear L365 L366
  constraint collinear L366 L367
  constraint collinear L368 L369
  constraint collinear L369 L370
  constraint collinear L371 L372
  constraint collinear L372 L373
  constraint collinear L374 L375
  constraint collinear L375 L376
  constraint collinear L377 L378
  constraint collinear L378 L379
  constraint collinear L380 L382
  constraint collinear L381 L384
  constraint collinear L382 L383
  constraint collinear L384 L385
  constraint collinear L386 L390
  constraint collinear L387 L388
  constraint collinear L388 L389
  constraint collinear L390 L391
  constraint collinear L392 L394
  constraint collinear L393 L396
  constraint collinear L394 L395
  constraint collinear L396 L397
  constraint collinear L398 L402
  constraint collinear L399 L400
  constraint collinear L400 L401
  constraint collinear L402 L403
  constraint collinear L404 L408
  constraint collinear L405 L406
  constraint collinear L406 L407
  constraint collinear L408 L409
  constraint collinear L410 L417
  constraint collinear L411 L415
  constraint collinear L412 L413
  constraint collinear L413 L414
  constraint collinear L415 L416
  constraint collinear L417 L418
  constraint collinear L419 L420
  constraint collinear L420 L421
  constraint collinear L422 L423
  constraint collinear L423 L424
  constraint collinear L425 L426
  constraint collinear L426 L427
  constraint collinear L428 L429
  constraint collinear L429 L430
  constraint collinear L431 L433
  constraint collinear L432 L435
  constraint collinear L433 L434
  constraint collinear L435 L436
  measures "d1" distance of L0.start L0.end
  measures "d2" distance of L0.start L2.end
  measures "d3" distance of L4.start L4.end
  measures "d4" distance of L3 L247
  measures "d9" distance of L7.end L7.start
  measures "d10" distance of L2 L8
  measures "d15" distance of L2 P0
  measures "d16" distance of L3 P0
  measures "d17" distance of L2 P1
  measures "d18" distance of L1 P1